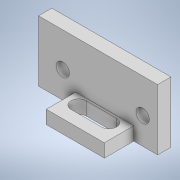
# Autodesk Inventor part: USB_C_Mount_Only
Saved by Autodesk Inventor 2021 (Build 250183000, 183)
## iProperties
Created: 2021-04-21
Part Number: USB_C_Mount_Only
Material: Generic
Document SubType Name: Modeling
Designer: Patrick
Density: 1 g/cm^3
Appearance: Default
Author: Patrick
Autodesk Inventor part; units mm, degrees
ref_plane "YZ Plane" through (0, 0, 0) normal (1, 0, 0) x (0, 1, 0)
ref_plane "XZ Plane" through (0, 0, 0) normal (0, 1, 0) x (-1, 0, 0)
ref_plane "XY Plane" through (0, 0, 0) normal (0, 0, 1) x (1, 0, 0)
sketch "Sketch1" plane through (0, 0, 0) normal (0, 1, 0) x (-1, 0, 0)
  line L0 (0, 0) -> (11.5488, 0)
  line L1 (0, 0) -> (5.8, 0)
  circle A0 centre (0, 1.45) radius 1.45
  circle A1 centre (5.8, 1.45) radius 1.45
  line L2 (5.8, 2.9) -> (0, 2.9)
  circle A2 centre (5.8, 1.45) radius 1.45
  circle A3 centre (0, 1.45) radius 1.45
  line L3 (0, 0) -> (5.8, 0)
  line L4 (0, 2.9) -> (5.8, 2.9)
  line L5 (8.1871, 5.226) -> (-2.892, 5.226)
  line L6 (-2.892, 5.226) -> (-2.892, -2.9279)
  line L7 (-2.892, -2.9279) -> (8.1871, -2.9279)
  line L8 (8.1871, -2.9279) -> (8.1871, 5.226)
  point P0 (5.8, 0)
  constraints: 18 end point, 5 tangent, 4 centre point, 4 equal length, 2 coincident, 2 concentric, 2 horizontal, 1 perpendicular
extrude "Extrusion1" add sketch "Sketch1" along normal blind 2.54
sketch "Sketch2" plane through (2.892, 0, -2.9279) normal (0, 0, -1) x (-1, 0, 0)
  line L0 (0, 0) -> (11.0791, 0)
  line L1 (11.0791, 0) -> (11.0791, 13.97)
  line L2 (11.0791, 13.97) -> (0, 13.97)
  line L3 (0, 13.97) -> (0, 0)
  circle A0 centre (13.5418, 5.08) radius 1.27
  circle A1 centre (-1.6982, 5.08) radius 1.27
  line L4 (8.692, 0) -> (2.892, 0) projected
  line L5 (2.892, 0) -> (8.692, 0) projected
  line L6 (6.1758, 0) -> (6.1758, 1.3937)
  line L7 (0, 2.54) -> (11.0791, 2.54) projected
  line L8 (-4.5494, 0) -> (18.1858, 0)
  line L9 (18.1858, 0) -> (18.1858, 11.6287)
  line L10 (18.1858, 11.6287) -> (-4.5494, 11.6287)
  line L11 (-4.5494, 11.6287) -> (-4.5494, 0)
  dimension "d2" = 13.97
  dimension "d3" = 2.54
  dimension "d4" = 2.54
  dimension "d5" = 15.24
  dimension "d6" = 7.366
  dimension "d7" = 2.54
  dimension "d8" = 2.54
  constraints: 18 end point, 4 parallel, 3 perpendicular, 2 centre point, 2 horizontal, 1 point on line
  measures "d2" distance of L0.end L1.end
  measures "d3" diameter of A0
  measures "d4" diameter of A1
  measures "d5" distance of A0.centre A1.centre
  measures "d6" distance from line of L6 A0.centre
  measures "d7" distance from line of L7 A1.centre
  measures "d8" distance from line of A0.centre L7
extrude "Extrusion2" add sketch "Sketch2" against normal blind 2.54 contours L8 L11 L10 L3 | L3 L10 L1 L7 | L1 L10 L9 L8
body "Solid1"
